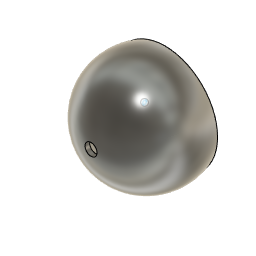
eye (Autodesk Fusion 360 design; units mm, degrees)
Autodesk Fusion 360 part; units mm, degrees
sketch "Esquisse1" plane through (0, 0, 0) normal (0, 0, 1) x (1, 0, 0)
sphere "SpherePrimitive1" add diameter 120 placed x (1, 0, 0) y (0, 1, 0) z (0, 0, 1) at (0, 0, 0) makes body 1
sketch "Esquisse2" plane through (0, 0, 0) normal (0, 0, 1) x (1, 0, 0)
  line L0 (100, 0) -> (140, 0)
  line L1 (100, 0) -> (100, 30)
  line L2 (100, 30) -> (140, 30)
  line L3 (140, 30) -> (140, 0)
  dimension "d2" = 40
  dimension "d3" = 30
  dimension "d4" = 40
  constraint horizontal L0
  constraint perpendicular L0 L1
  constraint perpendicular L1 L2
  measures "d2" distance of L0.start L0.end
  measures "d3" distance of L0.start L1.end
  measures "d4" distance of L1.end L2.end
sphere "SpherePrimitive2" add diameter 80 placed x (1, 0, 0) y (0, 1, 0) z (0, 0, 1) at (0, -100, 0) separate body makes body 2
delete_face "DeleteFace1" 1 faces at (37.923, -90.5447, -8.5115) on bodies 2
sketch "Esquisse4" plane through (0, 0, 0) normal (0, 0, 1) x (1, 0, 0)
  circle A0 centre (0, 60) radius 40
  dimension "d8" = 80
  measures "d8" diameter of A0
sphere "SpherePrimitive3" cut diameter 80 placed x (1, 0, 0) y (0, 1, 0) z (0, 0, 1) at (0, 60, 0) bodies 1
sketch "Esquisse5" plane through (0, 0, 0) normal (0, 0, 1) x (1, 0, 0)
  circle A0 centre (0, 0) radius 58.75
  dimension "d10" = 117.5
  constraint coincident A0.centre origin
  measures "d10" diameter of A0
sphere "SpherePrimitive4" cut diameter 110 placed x (1, 0, 0) y (0, 1, 0) z (0, 0, 1) at (0, 0, 0) bodies 1
sphere "SpherePrimitive5" add diameter 7.344 placed x (0, 1, 0) y (0, 0, 1) z (1, 0, 0) at (0, -775, 180) separate body makes body 3
delete_face "DeleteFace2" 1 faces at (3.4813, -775.868, 179.2186) on bodies 3
sketch "Esquisse7" plane through (0, 0, 0) normal (0, 0, 1) x (1, 0, 0)
  circle A0 centre (0, -60) radius 7.5
  dimension "d15" = 15
  measures "d15" diameter of A0
sketch "Esquisse9" plane through (0, 0, 0) normal (1, 0, 0) x (0, 1, 0)
  line L0 (0, 10) -> (0, 60)
  line L1 (0, 0) -> (-20, 0)
  line L2 (-20, 0) -> (-20, 20)
  line L3 (-20, 20) -> (0, 20)
  line L4 (0, 20) -> (0, 0)
  dimension "d19" = 20
  constraint vertical L0
  constraint horizontal L1
  constraint vertical L2
  constraint horizontal L3
  constraint vertical L4
  constraint coincident L1.start L4.end
  measures "d19" distance of L1.start L1.end
extrude "Extrusion2" add sketch "Esquisse9" along normal up to surface end surface at (41.9123, 33.5432, -11.9671) on bodies 1 bodies 1
sketch "Esquisse10" plane through (0, 0, 0) normal (0, 1, 0) x (-1, 0, 0)
  arc A0 (-51.2348, 20) -> (-55, 0) centre (0, 0) ccw
  line L0 (-55, 0) -> (0, 0)
  line L1 (0, 0) -> (0, 20)
  line L2 (0, 20) -> (-51.2348, 20)
  line L3 (0, 20) -> (-5, 20)
  line L4 (-5, 20) -> (-5, 0)
  line L5 (-5, 0) -> (0, 0)
  line L6 (0, 0) -> (0, 20)
  dimension "d22" = 5
  constraint horizontal L3
  constraint vertical L4
  constraint horizontal L5
  constraint vertical L6
  constraint coincident L1.end L2.start
  constraint coincident L5 A0.centre
  measures "d22" distance of L4 L6
extrude "Extrusion3" cut sketch "Esquisse10" against normal blind 29 contours L0 L1 L2 L3 L4 L5 L6 bodies 1
chamfer "Chanfrein1" distance 8 angle 45 4 edges at (54.0505, 0, 10.1757) (54.0505, -10.1757, 0) (50.2083, -10.2044, 20) (50.2083, -20, 10.2044) on bodies 1
sketch "Esquisse11" plane through (0, 0, 0) normal (1, 0, 0) x (0, 1, 0)
extrude "Extrusion4" cut 1 faces at (5, -6.6667, 13.3333) along direction (1, 0, 0) blind 5 on bodies 1 bodies 1
ref_plane "Plan de construction1" through (-5, 20, -5) normal (0, 1, 0) x (1, 0, 0)
split "Scinder1" by plane through (-5, 20, -5) normal (0, 1, 0) bodies 1 makes body 4 at (40.7785, 40.3525, 17.5724)
ref_plane "Plan de construction2" through (10, -10, 10) normal (-1, 0, 0) x (0, 0, 1)
sketch "Esquisse13" plane through (0, 0, 0) normal (1, 0, 0) x (0, 1, 0)
  circle A0 centre (-2, 15) radius 2
  dimension "d30" = 4
  measures "d30" diameter of A0
sketch "Esquisse14" plane through (0, 0, 0) normal (0, 1, 0) x (-1, 0, 0)
  line L0 (-10, 0) -> (-10, 20)
  line L1 (-10, 20) -> (-42.5323, 20)
  arc A0 (-42.5323, 20) -> (-47, 0) centre (0, 0) ccw
  line L2 (-47, 0) -> (-10, 0)
  circle A1 centre (-34, 13) radius 2.25
  circle A2 centre (-15, 13) radius 2.25
  line L3 (-10, 13) -> (-74.0312, 13) construction
  dimension "d31" = 4.5
  dimension "d32" = 4.5
  dimension "d33" = 19
  dimension "d34" = 13
  dimension "d35" = 5
  constraint coincident L0 L3.start
  constraint parallel L1 L3
  constraint coincident A1.centre L3
  constraint coincident A2.centre L3
  measures "d31" diameter of A1
  measures "d32" diameter of A2
  measures "d33" distance of A1.centre A2.centre
  measures "d34" distance of L2 L3
  measures "d35" distance of L0 A2.centre
extrude "Extrusion5" cut sketch "Esquisse14" against normal blind 29 contours A1 | A2 bodies 1
cylinder "CylindrePrimitive1" cut diameter 13 height -130 placed x (1, 0, 0) y (0, 0, -1) z (0, 1, 0) at (0, 0, 0) bodies 1
hidden bodies 4
